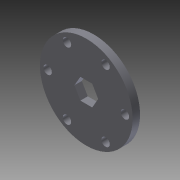
# Autodesk Inventor part: Custom Hex Hub
Saved by Autodesk Inventor 2014 SP1 (Build 180222100, 222)
## iProperties
Created: 2012-01-30
Part Number: Custom Hex Hub
Material: Steel
Document SubType Name: Modeling
Designer: Moses
Mass: 82.5117 g
Surface Area: 60.6656 cm^2
Volume: 10.511 cm^3
Density: 7.85 g/cm^3
Appearance: Steel
Author: Moses
Autodesk Inventor part; units mm, degrees
ref_plane "YZ Plane" through (0, 0, 0) normal (1, 0, 0) x (0, 1, 0)
ref_plane "XZ Plane" through (0, 0, 0) normal (0, 1, 0) x (-1, 0, 0)
ref_plane "XY Plane" through (0, 0, 0) normal (0, 0, 1) x (1, 0, 0)
sketch "Sketch1" plane through (0, 0, 0) normal (0, 0, 1) x (1, 0, 0)
  circle A0 centre (0, 0) radius 28.575
  circle A1 centre (-23.8125, 0) radius 2.5908
  line L0 (7.3323, 0) -> (3.6662, -6.35)
  line L1 (3.6662, -6.35) -> (-3.6662, -6.35)
  line L2 (-3.6662, -6.35) -> (-7.3323, 0)
  line L3 (-7.3323, 0) -> (-3.6662, 6.35)
  line L4 (-3.6662, 6.35) -> (3.6662, 6.35)
  line L5 (3.6662, 6.35) -> (7.3323, 0)
  line L6 (-23.8125, 0) -> (0, 0) construction
  circle A2 centre (-11.9063, 20.6222) radius 2.5908
  circle A3 centre (11.9062, 20.6222) radius 2.5908
  circle A4 centre (23.8125, 0) radius 2.5908
  circle A5 centre (11.9063, -20.6222) radius 2.5908
  circle A6 centre (-11.9062, -20.6222) radius 2.5908
  dimension "d0" = 57.15
  dimension "d1" = 5.1816
  dimension "d2" = 12.7
  dimension "d3" = 23.8125
  dimension "d6" = 360
  constraints: 14 end point, 7 centre point, 2 coincident, 1 horizontal, 1 parallel, 26 other
  measures "d0" diameter of A0
  measures "d1" diameter of A1
  measures "d2" distance between parallel lines of L1 L4
  measures "d3" distance of L6.start L6.end
extrude "Extrusion1" add sketch "Sketch1" along normal blind 4.572
body "Solid1"
